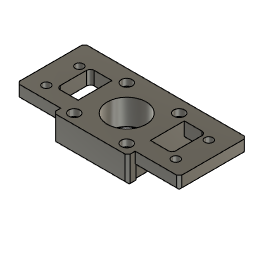
Z#motor_holder (Autodesk Fusion 360 design; units mm, degrees)
Autodesk Fusion 360 part; units mm, degrees
sketch "Sketch1" plane through (0, 0, 0) normal (0, 0, 1) x (1, 0, 0)
  line L0 (0, 0) -> (96, 0)
  line L1 (96, 0) -> (96, 40)
  line L2 (96, 40) -> (0, 40)
  line L3 (0, 40) -> (0, 0)
  dimension "d1" = 96
  dimension "d2" = 40
  constraint horizontal L0
  constraint vertical L1
  constraint horizontal L2
  constraint vertical L3
  constraint coincident L0.start L3.end
  measures "d1" distance of L0.start L0.end
  measures "d2" distance of L0.start L2.end
extrude "Extrude1" add sketch "Sketch1" along normal blind 6
sketch "Sketch2" plane through (0, 0, 6) normal (0, 0, 1) x (-1, 0, 0)
  line L0 (0, -40) -> (0, 0)
  line L1 (0, 0) -> (-96, 0)
  line L2 (-96, 0) -> (-96, -40)
  line L3 (-96, -40) -> (0, -40)
  line L4 (0, 0) -> (0, -7.5)
  line L5 (0, -7.5) -> (-10, -7.5)
  line L6 (0, -40) -> (0, -27)
  line L7 (0, -27) -> (-10, -27)
  line L8 (-96, 0) -> (-96, -8)
  line L9 (-96, -40) -> (-96, -27.5)
  line L10 (-96, -27.5) -> (-86, -27.5)
  line L11 (-96, -8) -> (-86, -8)
  circle A0 centre (-86, -8) radius 2.1
  circle A1 centre (-86, -27.5) radius 2.1
  circle A2 centre (-10, -27) radius 2.1
  circle A3 centre (-10, -7.5) radius 2.1
  dimension "d5" = 7.5
  dimension "d6" = 10
  dimension "d7" = 13
  dimension "d8" = 10
  dimension "d9" = 8
  dimension "d10" = 12.5
  dimension "d11" = 10
  dimension "d12" = 10
  dimension "d13" = 4.2
  dimension "d14" = 4.2
  dimension "d15" = 4.2
  dimension "d16" = 4.2
  constraint coincident L0.end L1.start
  constraint perpendicular L1 L4
  constraint perpendicular L4 L5
  constraint coincident L0.start L3.end
  constraint perpendicular L3 L6
  constraint perpendicular L6 L7
  constraint coincident L1.end L2.start
  constraint perpendicular L1 L8
  constraint coincident L2.end L3.start
  constraint perpendicular L3 L9
  constraint perpendicular L9 L10
  constraint perpendicular L2 L11
  constraint coincident L11.end A0.centre
  constraint coincident L10.end A1.centre
  constraint coincident L7.end A2.centre
  constraint coincident L5.end A3.centre
  measures "d5" distance of L0.end L4.end
  measures "d6" distance of L4.end L5.end
  measures "d7" distance of L0.start L6.end
  measures "d8" distance of L6.end L7.end
  measures "d9" distance of L1.end L8.end
  measures "d10" distance of L2.end L9.end
  measures "d11" distance of L9.end L10.end
  measures "d12" distance of L8.end L11.end
  measures "d13" diameter of A0
  measures "d14" diameter of A1
  measures "d15" diameter of A2
  measures "d16" diameter of A3
extrude "Extrude2" cut sketch "Sketch2" against normal blind 6 contours A0 | A1 | A2 | A3
extrude "Extrude3" add 1 faces at (36.0022, 14.373, 6) along direction (0, 0, 1) blind 2
sketch "Sketch3" plane through (0, 0, 8) normal (0, 0, 1) x (-1, 0, 0)
  circle A0 centre (-10, -27) radius 2.1
  circle A1 centre (-86, -27.5) radius 2.1
  circle A2 centre (-10, -7.5) radius 2.1
  circle A3 centre (-86, -8) radius 2.1
  line L0 (0, -40) -> (0, 0)
  line L1 (0, 0) -> (-96, 0)
  line L2 (-96, 0) -> (-96, -40)
  line L3 (-96, -40) -> (0, -40)
  line L4 (-48, -40) -> (-48, -17)
  circle A4 centre (-48, -17) radius 3
  dimension "d21" = 23
  dimension "d22" = 6
  constraint midpoint L3 L4.start
  constraint perpendicular L3 L4
  constraint coincident L4.end A4.centre
  measures "d21" distance of L4.start L4.end
  measures "d22" diameter of A4
extrude "Extrude4" cut sketch "Sketch3" against normal blind 50 contours A4
sketch "Sketch4" plane through (0, 0, 8) normal (0, 0, 1) x (-1, 0, 0)
  circle A0 centre (-48, -17) radius 3
  circle A1 centre (-10, -27) radius 2.1
  circle A2 centre (-86, -27.5) radius 2.1
  circle A3 centre (-10, -7.5) radius 2.1
  circle A4 centre (-86, -8) radius 2.1
  line L0 (0, -40) -> (0, 0)
  line L1 (0, 0) -> (-96, 0)
  line L2 (-96, 0) -> (-96, -40)
  line L3 (-96, -40) -> (0, -40)
  line L4 (-63.5, -17) -> (-63.5, -32.5)
  line L5 (-63.5, -17) -> (-63.5, -1.5)
  line L6 (-48, -32.5) -> (-32.5, -32.5)
  line L7 (-32.5, -32.5) -> (-32.5, -1.5)
  circle A5 centre (-32.5, -1.5) radius 1.6
  circle A6 centre (-63.5, -1.5) radius 1.6
  circle A7 centre (-63.5, -32.5) radius 1.6
  circle A8 centre (-32.5, -32.5) radius 1.6
  dimension "d28" = 15.5
  dimension "d29" = 31
  dimension "d30" = 3.2
  dimension "d31" = 3.2
  dimension "d32" = 3.2
  dimension "d33" = 3.2
  constraint perpendicular L6 L7
  constraint coincident L7.end A5.centre
  constraint coincident L5.end A6.centre
  constraint coincident L4.end A7.centre
  constraint coincident L6.end L7.start
  measures "d28" distance of L6.start L6.end
  measures "d29" distance of L6.end L7.end
  measures "d30" diameter of A5
  measures "d31" diameter of A6
  measures "d32" diameter of A7
  measures "d33" diameter of A8
sketch "Sketch5" plane through (0, 0, 0) normal (0, -1, 0) x (1, 0, 0)
  line L0 (0, 0) -> (96, 0)
  line L1 (96, 0) -> (96, 8)
  line L2 (96, 8) -> (0, 8)
  line L3 (0, 8) -> (0, 0)
  line L4 (48, 8) -> (29, 8)
  line L5 (48, 8) -> (67, 8)
  line L6 (29, 8) -> (67, 8)
  line L7 (67, 8) -> (67, 0)
  line L8 (67, 0) -> (29, 0)
  line L9 (29, 0) -> (29, 8)
  constraint midpoint L2 L4.start
  constraint coincident L2 L4.end
  constraint parallel L2 L4
  constraint coincident L2 L5.end
  constraint parallel L2 L5
  constraint horizontal L6
  constraint vertical L7
  constraint horizontal L8
  constraint vertical L9
  constraint coincident L0 L7.end
extrude "Extrude5" add sketch "Sketch5" along normal blind 1.5 contours L0 L2 L4 L5 L6 L7 L8 L9
extrude "Extrude6" cut sketch "Sketch4" against normal blind 50 contours L1 A5 | L1 A6 | L6 L7 A8 | L6 L7 A8 | A7 picked at (-32.9612, -1.8296) picked at (-63.2941, -1.1119)
sketch "Sketch6" plane through (0, 0, 8) normal (0, 0, 1) x (-1, 0, 0)
  line L0 (-64.0568, 0) -> (-62.9432, 0)
  arc A0 (-64.0568, 0) -> (-62.9432, 0) centre (-63.5, -1.5) ccw
  line L1 (-33.0568, 0) -> (-31.9432, 0)
  arc A1 (-33.0568, 0) -> (-31.9432, 0) centre (-32.5, -1.5) ccw
  circle A2 centre (-63.5, -32.5) radius 1.6
  circle A3 centre (-32.5, -32.5) radius 1.6
  circle A4 centre (-48, -17) radius 3
  circle A5 centre (-10, -27) radius 2.1
  circle A6 centre (-86, -27.5) radius 2.1
  circle A7 centre (-10, -7.5) radius 2.1
  circle A8 centre (-86, -8) radius 2.1
  line L2 (0, -40) -> (0, 0)
  line L3 (0, 0) -> (-29, 0)
  line L4 (-29, 0) -> (-29, 1.5)
  line L5 (-29, 1.5) -> (-67, 1.5)
  line L6 (-67, 1.5) -> (-67, 0)
  line L7 (-67, 0) -> (-96, 0)
  line L8 (-96, 0) -> (-96, -40)
  line L9 (-96, -40) -> (0, -40)
  circle A9 centre (-48, -17) radius 11.5
  dimension "d38" = 23
  constraint concentric A4 A9
  measures "d38" diameter of A9
extrude "Extrude7" cut sketch "Sketch6" against normal blind 2.5 contours A9
extrude "Extrude8" add 1 faces at (41.6667, -1.5, 5.3333) along direction (0, -1, 0) blind 1
fillet "Fillet1" radius 1 1 edges at (48, -2.5, 0)
sketch "Sketch7" plane through (0, 0, 0) normal (0, 0, -1) x (1, 0, 0)
  line L0 (67, 1.5) -> (29, 1.5)
  line L1 (29, 1.5) -> (29, 0)
  line L2 (29, 0) -> (0, 0)
  line L3 (0, 0) -> (0, -40)
  line L4 (0, -40) -> (96, -40)
  line L5 (96, -40) -> (96, 0)
  line L6 (96, 0) -> (67, 0)
  line L7 (67, 0) -> (67, 1.5)
  line L8 (62.9432, 0) -> (64.0568, 0)
  arc A0 (62.9432, 0) -> (64.0568, 0) centre (63.5, -1.5) ccw
  line L9 (31.9432, 0) -> (33.0568, 0)
  arc A1 (31.9432, 0) -> (33.0568, 0) centre (32.5, -1.5) ccw
  circle A2 centre (63.5, -32.5) radius 1.6
  circle A3 centre (32.5, -32.5) radius 1.6
  circle A4 centre (48, -17) radius 3
  circle A5 centre (10, -27) radius 2.1
  circle A6 centre (86, -27.5) radius 2.1
  circle A7 centre (10, -7.5) radius 2.1
  circle A8 centre (86, -8) radius 2.1
  circle A9 centre (32.5, -32.5) radius 2.6
  circle A10 centre (63.5, -32.5) radius 2.6
  circle A11 centre (63.5, -1.5) radius 2.6
  circle A12 centre (32.5, -1.5) radius 2.6
  dimension "d44" = 5.2
  dimension "d45" = 5.2
  dimension "d46" = 5.2
  dimension "d47" = 5.2
  constraint concentric A3 A9
  constraint concentric A2 A10
  constraint concentric A0 A11
  constraint concentric A1 A12
  measures "d44" diameter of A9
  measures "d45" diameter of A10
  measures "d46" diameter of A11
  measures "d47" diameter of A12
extrude "Extrude9" cut sketch "Sketch7" against normal blind 3.5 contours A9 | A10 | A11 | A12
extrude "Extrude10" add 1 faces at (29, -0.8333, 3) along direction (-1, 0, 0) blind 3
extrude "Extrude11" add 1 faces at (67, -0.8333, 3) along direction (1, 0, 0) blind 3
fillet "Fillet2" radius 1 3 edges at (70, -2.5, 4.5) (70, -2.2071, 0.2929) (70, -0.75, 0)
fillet "Fillet3" radius 1 3 edges at (26, -0.75, 0) (26, -2.2071, 0.2929) (26, -2.5, 4.5)
chamfer "Chamfer1" distance 1.5 angle 45 2 edges at (82.5, 0, 0) (13.5, 0, 0)
chamfer "Chamfer2" distance 1.5 angle 45 3 edges at (48, 40, 0) (0, 20.75, 0) (96, 20.75, 0)
chamfer "Chamfer3" distance 1.5 angle 45 2 edges at (96, 40, 4.75) (0, 40, 4.75)
chamfer "Chamfer4" distance 1.5 angle 45 2 edges at (96, 0, 4.75) (0, 0, 4.75)
extrude "Extrude12" cut sketch "Sketch4" against normal blind 50 contours L1 A6 picked at (-63.6129, 0.0213)
extrude "Extrude13" cut sketch "Sketch4" against normal blind 50 contours L1 A5 picked at (-32.6129, 0.0213)
sketch "Sketch9" plane through (0, 0, 5.5) normal (0, 0, 1) x (-1, 0, 0)
  circle A0 centre (-48, -17) radius 3
  circle A1 centre (-48, -17) radius 11.5
  circle A2 centre (-48, -17) radius 11.5
  constraint concentric A0 A2
sketch "Sketch10" plane through (0, 0, 0) normal (0, 0, -1) x (1, 0, 0)
  circle A0 centre (32.5, -1.5) radius 2.6
  circle A1 centre (32.5, -32.5) radius 2.6
  circle A2 centre (63.5, -1.5) radius 2.6
  circle A3 centre (63.5, -32.5) radius 2.6
  circle A4 centre (48, -17) radius 3
  circle A5 centre (10, -27) radius 2.1
  circle A6 centre (86, -27.5) radius 2.1
  circle A7 centre (10, -7.5) radius 2.1
  circle A8 centre (86, -8) radius 2.1
  line L0 (1.5, -1.5) -> (1.5, -38.5)
  line L1 (1.5, -38.5) -> (94.5, -38.5)
  line L2 (94.5, -38.5) -> (94.5, -1.5)
  line L3 (94.5, -1.5) -> (69, -1.5)
  line L4 (69, -1.5) -> (69, 1.5)
  line L5 (69, 1.5) -> (27, 1.5)
  line L6 (27, 1.5) -> (27, -1.5)
  line L7 (27, -1.5) -> (1.5, -1.5)
  circle A9 centre (48, -17) radius 11.5
  dimension "d64" = 23
  constraint concentric A4 A9
  measures "d64" diameter of A9
extrude "Extrude14" cut sketch "Sketch10" against normal blind 2.5 contours A9
extrude "Extrude15" add sketch "Sketch9" along normal blind 2.5
extrude "Extrude16" add 4 faces at (64.508, 3.5241, 3.5) (64.5166, 34.5192, 3.5) (34.751, 32.7087, 3.5) (34.7569, 1.6391, 3.5) along direction (0, 0, -1) blind 3.5
sketch "Sketch11" plane through (0, 0, 8) normal (0, 0, 1) x (-1, 0, 0)
  circle A0 centre (-48, -17) radius 3
  circle A1 centre (-32.5, -1.5) radius 1.6
  circle A2 centre (-63.5, -1.5) radius 1.6
  circle A3 centre (-63.5, -32.5) radius 1.6
  circle A4 centre (-32.5, -32.5) radius 1.6
  circle A5 centre (-10, -27) radius 2.1
  circle A6 centre (-86, -27.5) radius 2.1
  circle A7 centre (-10, -7.5) radius 2.1
  circle A8 centre (-86, -8) radius 2.1
  line L0 (0, -1.5) -> (-1.5, 0)
  line L1 (-1.5, 0) -> (-26, 0)
  line L2 (-26, 0) -> (-26, 1.5)
  arc A9 (-26, 1.5) -> (-27, 2.5) centre (-27, 1.5) ccw
  line L3 (-27, 2.5) -> (-69, 2.5)
  arc A10 (-69, 2.5) -> (-70, 1.5) centre (-69, 1.5) ccw
  line L4 (-70, 1.5) -> (-70, 0)
  line L5 (-70, 0) -> (-94.5, 0)
  line L6 (-94.5, 0) -> (-96, -1.5)
  line L7 (-96, -1.5) -> (-96, -38.5)
  line L8 (-96, -38.5) -> (-94.5, -40)
  line L9 (-94.5, -40) -> (-1.5, -40)
  line L10 (-1.5, -40) -> (0, -38.5)
  line L11 (0, -38.5) -> (0, -1.5)
  circle A11 centre (-63.5, -32.5) radius 3.25
  circle A12 centre (-63.5, -1.5) radius 3.25
  circle A13 centre (-32.5, -1.5) radius 3.25
  circle A14 centre (-32.5, -32.5) radius 3.25
  dimension "d71" = 6.5
  dimension "d72" = 6.5
  dimension "d73" = 6.5
  dimension "d74" = 6.5
  constraint concentric A3 A11
  constraint concentric A2 A12
  constraint concentric A1 A13
  constraint concentric A4 A14
  measures "d71" diameter of A11
  measures "d72" diameter of A12
  measures "d73" diameter of A13
  measures "d74" diameter of A14
extrude "Extrude17" cut sketch "Sketch11" against normal blind 4 contours A11 | A12 | A13 | A14
sketch "Sketch12" plane through (0, 0, 0) normal (0, 0, -1) x (1, 0, 0)
  circle A0 centre (32.5, -1.5) radius 1.6
  circle A1 centre (63.5, -32.5) radius 1.6
  circle A2 centre (63.5, -1.5) radius 1.6
  circle A3 centre (32.5, -32.5) radius 1.6
  circle A4 centre (48, -17) radius 11.5
  circle A5 centre (10, -27) radius 2.1
  circle A6 centre (86, -27.5) radius 2.1
  circle A7 centre (10, -7.5) radius 2.1
  circle A8 centre (86, -8) radius 2.1
  line L0 (1.5, -1.5) -> (1.5, -38.5)
  line L1 (1.5, -38.5) -> (94.5, -38.5)
  line L2 (94.5, -38.5) -> (94.5, -1.5)
  line L3 (94.5, -1.5) -> (69, -1.5)
  line L4 (69, -1.5) -> (69, 1.5)
  line L5 (69, 1.5) -> (27, 1.5)
  line L6 (27, 1.5) -> (27, -1.5)
  line L7 (27, -1.5) -> (1.5, -1.5)
  line L8 (27, 1.5) -> (69, 1.5)
  line L9 (69, 1.5) -> (69, -38.5)
  line L10 (69, -38.5) -> (27, -38.5)
  line L11 (27, -38.5) -> (27, 1.5)
  constraint horizontal L8
  constraint vertical L9
  constraint horizontal L10
  constraint vertical L11
  constraint coincident L1 L9.end
  constraint coincident L5.end L6.start
extrude "Extrude18" add sketch "Sketch12" along normal blind 8 contours L1 L4 L5 L6 L8 L9 L10 L11
extrude "Extrude19" cut 1 faces at (56.6239, 17.5713, 2.5) along direction (0, 0, 1) blind 32
delete_face "DeleteFace1" 1 faces at (69.1305, -2.3276, 0.4541)
sketch "Sketch13" plane through (0, 0, -8) normal (0, 0, -1) x (1, 0, 0)
  circle A0 centre (32.5, -32.5) radius 1.6
  circle A1 centre (63.5, -1.5) radius 1.6
  circle A2 centre (63.5, -32.5) radius 1.6
  circle A3 centre (48, -17) radius 11.5
  circle A4 centre (32.5, -1.5) radius 1.6
  line L0 (27, -38.5) -> (69, -38.5)
  line L1 (69, -38.5) -> (69, 1.5)
  line L2 (69, 1.5) -> (27, 1.5)
  line L3 (27, 1.5) -> (27, -38.5)
  line L4 (26, -1.5) -> (70, -1.5)
  line L5 (70, -1.5) -> (70, 2.5)
  line L6 (70, 2.5) -> (26, 2.5)
  line L7 (26, 2.5) -> (26, -1.5)
  constraint horizontal L4
  constraint vertical L5
  constraint horizontal L6
  constraint vertical L7
extrude "Extrude20" add sketch "Sketch13" against normal blind 16 contours L1 L2 L3 L4 L5 L6 L7
extrude "Extrude21" cut sketch "Sketch11" against normal blind 4 contours A13
extrude "Extrude22" cut sketch "Sketch11" against normal blind 4 contours A12
extrude "Extrude23" add 1 faces at (55, -2.5, -2.6667) along direction (0, -1, 0) blind 2
delete_face "DeleteFace2" 1 faces at (95.5, 39, 5.8333)
delete_face "DeleteFace3" 1 faces at (95.5, 1, 3.6667)
delete_face "DeleteFace4" 1 faces at (1, 39.5, 5.8333)
chamfer "Chamfer5" distance 16 angle 45 1 edges at (96, 40, 4.75)
chamfer "Chamfer6" distance 16 angle 45 1 edges at (0, 40, 4.75)
delete_face "DeleteFace5" 1 faces at (55, 39.5, 1)
chamfer "Chamfer7" distance 11 angle 45 1 edges at (96, 0, 4.75)
delete_face "DeleteFace6" 1 faces at (0.5, 1, 3.6667)
chamfer "Chamfer8" distance 11 angle 45 1 edges at (0, 0, 4.75)
delete_face "DeleteFace7" 1 faces at (95, 19.6667, 0.5)
delete_face "DeleteFace8" 1 faces at (1, 15.3333, 0.5)
chamfer "Chamfer9" distance 1.5 angle 45 1 edges at (70, -4.5, 0)
chamfer "Chamfer10" distance 1.5 angle 45 1 edges at (26, -4.5, 0)
chamfer "Chamfer11" distance 1.5 angle 45 1 edges at (27, 38.5, -4)
chamfer "Chamfer12" distance 1.5 angle 45 1 edges at (69, 38.5, -4)
chamfer "Chamfer13" distance 1 angle 45 1 edges at (70, 1.5, -4)
chamfer "Chamfer14" distance 1 angle 45 1 edges at (26, 1.5, -4)
chamfer "Chamfer15" distance 1 angle 45 1 edges at (27, 19.25, -8)
chamfer "Chamfer16" distance 1 angle 45 1 edges at (48, 38.5, -8)
chamfer "Chamfer17" distance 1 angle 45 1 edges at (69, 19.25, -8)
chamfer "Chamfer18" distance 2 angle 45 1 edges at (48, -4.5, -8)
chamfer "Chamfer19" distance 1 angle 45 2 edges at (70, -1, -8) (69, 1.5, -8)
chamfer "Chamfer20" distance 1 angle 45 2 edges at (26, -1, -8) (27, 1.5, -8)
sketch "Sketch14" plane through (0, 0, 8) normal (0, 0, 1) x (-1, 0, 0)
  line L0 (-26, 3) -> (-27.5, 4.5)
  line L1 (-27.5, 4.5) -> (-68.5, 4.5)
  line L2 (-68.5, 4.5) -> (-70, 3)
  line L3 (-70, 3) -> (-70, 0)
  line L4 (-70, 0) -> (-85, 0)
  line L5 (-85, 0) -> (-96, -11)
  line L6 (-96, -11) -> (-96, -24)
  line L7 (-96, -24) -> (-80, -40)
  line L8 (-80, -40) -> (-16, -40)
  line L9 (-16, -40) -> (0, -24)
  line L10 (0, -24) -> (0, -11)
  line L11 (0, -11) -> (-11, 0)
  line L12 (-11, 0) -> (-26, 0)
  line L13 (-26, 0) -> (-26, 3)
  circle A0 centre (-48, -17) radius 11.5
  circle A1 centre (-32.5, -32.5) radius 3.25
  circle A2 centre (-63.5, -32.5) radius 3.25
  circle A3 centre (-10, -27) radius 2.1
  circle A4 centre (-86, -27.5) radius 2.1
  circle A5 centre (-10, -7.5) radius 2.1
  circle A6 centre (-86, -8) radius 2.1
  circle A7 centre (-32.5, -1.5) radius 3.25
  circle A8 centre (-63.5, -1.5) radius 3.25
  circle A9 centre (-86, -8) radius 2.4
  circle A10 centre (-86, -27.5) radius 2.4
  circle A11 centre (-10, -27) radius 2.4
  circle A12 centre (-10, -7.5) radius 2.4
  dimension "d105" = 4.8
  dimension "d106" = 4.8
  dimension "d107" = 4.8
  dimension "d108" = 4.8
  constraint concentric A6 A9
  constraint concentric A4 A10
  constraint concentric A3 A11
  constraint concentric A5 A12
  measures "d105" diameter of A9
  measures "d106" diameter of A10
  measures "d107" diameter of A11
  measures "d108" diameter of A12
extrude "Extrude24" cut sketch "Sketch14" against normal blind 500 contours A9 | A10 | A11 | A12
sketch "Sketch15" plane through (0, 0, 0) normal (0, 0, -1) x (1, 0, 0)
  circle A0 centre (10, -7.5) radius 2.4
  circle A1 centre (86, -8) radius 2.4
  circle A2 centre (10, -27) radius 2.4
  circle A3 centre (86, -27.5) radius 2.4
  line L0 (0, -24) -> (16, -40)
  line L1 (16, -40) -> (80, -40)
  line L2 (80, -40) -> (96, -24)
  line L3 (96, -24) -> (96, -11)
  line L4 (96, -11) -> (86.5, -1.5)
  line L5 (86.5, -1.5) -> (69, -1.5)
  line L6 (69, -1.5) -> (69, -37)
  line L7 (69, -37) -> (67.5, -38.5)
  line L8 (67.5, -38.5) -> (28.5, -38.5)
  line L9 (28.5, -38.5) -> (27, -37)
  line L10 (27, -37) -> (27, -1.5)
  line L11 (27, -1.5) -> (9.5, -1.5)
  line L12 (9.5, -1.5) -> (0, -11)
  line L13 (0, -11) -> (0, -24)
  line L14 (0, -11) -> (0, 0)
  line L15 (0, 0) -> (11, 0)
  line L16 (11, 0) -> (0, -11)
  line L17 (16, -40) -> (0, -40)
  line L18 (0, -40) -> (0, -24)
  line L19 (96, -11) -> (96, 0)
  line L20 (96, 0) -> (85, 0)
  line L21 (85, 0) -> (96, -11)
  line L22 (96, -24) -> (96, -40)
  line L23 (96, -40) -> (80, -40)
  constraint coincident L12.end L13.start
  constraint coincident L14.end L15.start
  constraint perpendicular L14 L15
  constraint parallel L12 L16
  constraint coincident L0.end L1.start
  constraint parallel L1 L17
  constraint coincident L0.start L13.end
  constraint perpendicular L17 L18
  constraint coincident L3.end L4.start
  constraint perpendicular L5 L19
  constraint perpendicular L19 L20
  constraint parallel L4 L21
  constraint coincident L2.end L3.start
  constraint parallel L3 L22
  constraint coincident L1.end L2.start
extrude "Extrude25" add sketch "Sketch15" against normal blind 8 contours L0 L17 L18 | L12 L14 L15 L16 | L2 L22 L23 | L4 L19 L20 L21
sketch "Sketch16" plane through (0, 0, 0) normal (0, 0, -1) x (1, 0, 0)
  circle A0 centre (10, -7.5) radius 2.4
  circle A1 centre (86, -8) radius 2.4
  circle A2 centre (10, -27) radius 2.4
  circle A3 centre (86, -27.5) radius 2.4
  line L0 (0, -40) -> (80, -40)
  line L1 (80, -40) -> (96, -40)
  line L2 (96, -40) -> (96, 0)
  line L3 (96, 0) -> (85, 0)
  line L4 (85, 0) -> (86.5, -1.5)
  line L5 (86.5, -1.5) -> (69, -1.5)
  line L6 (69, -1.5) -> (69, -37)
  line L7 (69, -37) -> (67.5, -38.5)
  line L8 (67.5, -38.5) -> (28.5, -38.5)
  line L9 (28.5, -38.5) -> (27, -37)
  line L10 (27, -37) -> (27, -1.5)
  line L11 (27, -1.5) -> (9.5, -1.5)
  line L12 (9.5, -1.5) -> (11, 0)
  line L13 (11, 0) -> (0, 0)
  line L14 (0, 0) -> (0, -40)
  line L15 (0, -40) -> (96, -40)
  line L16 (96, -40) -> (96, -42)
  line L17 (96, -42) -> (0, -42)
  line L18 (0, -42) -> (0, -40)
  dimension "d113" = 2
  constraint horizontal L15
  constraint vertical L16
  constraint horizontal L17
  constraint vertical L18
  constraint coincident L0.start L14.end
  measures "d113" distance of L0.start L17.end
extrude "Extrude26" add sketch "Sketch16" against normal blind 8 contours L0 L1 L15 L16 L17 L18
extrude "Extrude27" cut 1 faces at (64, 42, 2.6667) along direction (0, -1, 0) blind 2
delete_face "DeleteFace9" 1 faces at (80.5, 1, 0.5)
chamfer "Chamfer21" distance 1.5 angle 45 1 edges at (83, 0, 0)
delete_face "DeleteFace10" 1 faces at (15.5, 0.6667, 0.8333)
chamfer "Chamfer22" distance 1.5 angle 45 1 edges at (13, 0, 0)
chamfer "Chamfer23" distance 1.5 angle 45 3 edges at (0, 20.75, 0) (48, 40, 0) (96, 20.75, 0)
chamfer "Chamfer24" distance 1.5 angle 45 2 edges at (0, 40, 4.75) (96, 40, 4.75)
chamfer "Chamfer25" distance 1.5 angle 45 1 edges at (0, 0, 4.75)
chamfer "Chamfer26" distance 1.5 angle 45 1 edges at (96, 0, 4.75)
sketch "Sketch17" plane through (0, 0, 0) normal (0, 0, -1) x (1, 0, 0)
  line L0 (94.5, -38.5) -> (94.5, -1.5)
  line L1 (94.5, -1.5) -> (69, -1.5)
  line L2 (69, -1.5) -> (69, -37)
  line L3 (69, -37) -> (67.5, -38.5)
  line L4 (67.5, -38.5) -> (94.5, -38.5)
  circle A0 centre (86, -27.5) radius 2.4
  circle A1 centre (86, -8) radius 2.4
  line L5 (81.75, -10) -> (69, -10)
  line L6 (81.75, -20) -> (81.75, -30)
  line L7 (69, -30) -> (81.75, -30)
  line L8 (81.75, -20) -> (81.75, -10)
  constraint coincident L2 L5.end
  constraint perpendicular L2 L5
  constraint perpendicular L5 L6
  constraint coincident L2 L7.start
  constraint perpendicular L5 L8
extrude "Extrude28" cut sketch "Sketch17" against normal blind 10 contours L2 L5 L6 L7 L8
sketch "Sketch18" plane through (0, 0, 0) normal (0, 0, -1) x (1, 0, 0)
  line L0 (1.5, -38.5) -> (28.5, -38.5)
  line L1 (28.5, -38.5) -> (27, -37)
  line L2 (27, -37) -> (27, -1.5)
  line L3 (27, -1.5) -> (1.5, -1.5)
  line L4 (1.5, -1.5) -> (1.5, -38.5)
  circle A0 centre (10, -27) radius 2.4
  circle A1 centre (10, -7.5) radius 2.4
  line L5 (27, -19.25) -> (14.25, -19.25)
  line L6 (14.25, -19.25) -> (14.25, -9.25)
  line L7 (14.25, -19.25) -> (14.25, -29.25)
  line L8 (14.25, -29.25) -> (27, -29.25)
  line L9 (14.25, -9.25) -> (27, -9.25)
  dimension "d128" = 12.75
  dimension "d129" = 10
  dimension "d130" = 10
  constraint midpoint L2 L5.start
  constraint perpendicular L2 L5
  constraint perpendicular L5 L6
  constraint perpendicular L5 L7
  constraint coincident L2 L8.end
  constraint perpendicular L2 L8
  constraint coincident L2 L9.end
  constraint perpendicular L2 L9
  measures "d128" distance of L5.start L5.end
  measures "d129" distance of L5.end L6.end
  measures "d130" distance of L5.end L7.end
extrude "Extrude29" cut sketch "Sketch18" against normal blind 100 contours L2 L5 L7 L8 | L2 L5 L6 L9
fillet "Fillet4" radius 2.25 1 edges at (14.25, 29.25, 4)
fillet "Fillet5" radius 2.25 1 edges at (14.25, 9.25, 4)
fillet "Fillet6" radius 2.25 1 edges at (81.75, 10, 4)
fillet "Fillet7" radius 2.25 1 edges at (81.75, 30, 4)
chamfer "Chamfer27" distance 1 angle 45 1 edges at (37.2782, 12.8414, -8)
delete_face "DeleteFace11" 1 faces at (68, 38, -2.3333)
delete_face "DeleteFace12" 1 faces at (55.1667, 38.1667, -7.3333)
delete_face "DeleteFace13" 1 faces at (28, 38, -5)
delete_face "DeleteFace14" 1 faces at (63.5, 39.0002, 0.4999)
extrude "Extrude30" add 1 faces at (54.6667, 38.5, -2.6667) along direction (0, 1, 0) blind 1.5
chamfer "Chamfer28" distance 1.5 angle 45 1 edges at (81.75, 40, 0)
chamfer "Chamfer29" distance 1.5 angle 45 1 edges at (14.25, 40, 0)
chamfer "Chamfer30" distance 1 angle 45 1 edges at (48, 40, -8)
chamfer "Chamfer31" distance 1 angle 45 1 edges at (69, 40, -2.75)
chamfer "Chamfer32" distance 1 angle 45 1 edges at (27, 40, -2.75)
equation "d3 = 3 mm + 3 mm"
